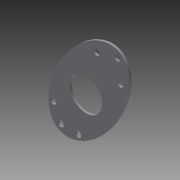
# Autodesk Inventor part: Bottom Hub Plate
Saved by Autodesk Inventor 2015 (Build 190159000, 159)
## iProperties
Created: 2015-01-24
Part Number: Bottom Hub Plate
Material: Generic
Document SubType Name: Modeling
Designer: Brian
Density: 1 g/cm^3
Appearance: Default
Author: Brian
Autodesk Inventor part; units mm, degrees
ref_plane "YZ Plane" through (0, 0, 0) normal (1, 0, 0) x (0, 1, 0)
ref_plane "XZ Plane" through (0, 0, 0) normal (0, 1, 0) x (-1, 0, 0)
ref_plane "XY Plane" through (0, 0, 0) normal (0, 0, 1) x (1, 0, 0)
sketch "Sketch1" plane through (0, 0, 0) normal (0, 0, 1) x (1, 0, 0)
  arc A0 (2.7781, 11.2277) -> (-2.7781, 11.2277) centre (0, 6.4158) ccw construction
  arc A1 (-2.7781, 11.2277) -> (-5.5562, 6.4158) centre (0, 6.4158) ccw construction
  arc A2 (-5.5562, 6.4158) -> (-2.7781, 1.604) centre (0, 6.4158) ccw construction
  arc A3 (-2.7781, 1.604) -> (2.7781, 1.604) centre (0, 6.4158) ccw construction
  arc A4 (2.7781, 1.604) -> (5.5562, 6.4158) centre (0, 6.4158) ccw construction
  arc A5 (5.5562, 6.4158) -> (2.7781, 11.2277) centre (0, 6.4158) ccw construction
  circle A6 centre (0, 6.4158) radius 3.1376 construction
  arc A7 (65.8645, 106.5408) -> (60.3083, 106.5408) centre (63.0864, 101.729) ccw construction
  arc A8 (60.3083, 106.5408) -> (57.5301, 101.729) centre (63.0864, 101.729) ccw construction
  arc A9 (57.5301, 101.729) -> (60.3083, 96.9171) centre (63.0864, 101.729) ccw construction
  arc A10 (60.3083, 96.9171) -> (65.8645, 96.9171) centre (63.0864, 101.729) ccw construction
  arc A11 (65.8645, 96.9171) -> (68.6426, 101.729) centre (63.0864, 101.729) ccw construction
  arc A12 (68.6426, 101.729) -> (65.8645, 106.5408) centre (63.0864, 101.729) ccw construction
  circle A13 centre (63.0864, 101.729) radius 3.1376 construction
  circle A14 centre (28.0384, 48.7772) radius 16.383 construction
  circle A15 centre (28.0384, 48.7772) radius 18.288
  circle A16 centre (0, 6.4158) radius 6.4158 construction
  circle A17 centre (63.0864, 101.729) radius 6.4158 construction
  circle A18 centre (63.0864, 101.729) radius 6.9238 construction
  circle A19 centre (0, 6.4158) radius 6.9238 construction
  circle A20 centre (0, 6.4158) radius 3.3916
  circle A21 centre (63.0864, 101.729) radius 3.3916
  circle A22 centre (28.0384, 48.7772) radius 38.1 construction
  line L0 (66.9079, 107.5026) -> (-3.8215, 0.6421) construction
  ellipse E0 centre (31.5432, 54.0724) end of major axis (-3.8215, 0.6421) minor radius 35.9584
  circle A23 centre (67.1501, 77.726) radius 3.302
  circle A24 centre (39.4038, 96.091) radius 3.302
  circle A25 centre (19.4364, 4.8439) radius 3.302
  circle A26 centre (-9.0413, 23.6929) radius 3.302
  line L1 (67.1501, 77.726) -> (53.277, 86.9085) construction
  line L2 (39.4038, 96.091) -> (53.277, 86.9085) construction
  line L3 (19.4364, 4.8439) -> (5.1975, 14.2684) construction
  line L4 (-9.0413, 23.6929) -> (5.1975, 14.2684) construction
  circle A27 centre (67.1501, 77.726) radius 10.5597 construction
  circle A28 centre (19.4364, 4.8439) radius 5.715 construction
  circle A29 centre (0, 6.4158) radius 13.7848 construction
  circle A30 centre (63.0864, 101.729) radius 13.7848 construction
  circle A31 centre (19.4364, 4.8439) radius 6.6675 construction
  point P0 (0, 0)
  point P1 (63.0864, 95.3131)
  point P2 (63.0864, 87.9441)
  point P3 (0, 20.2006)
  dimension "d3" = 0.508
  dimension "d4" = 0.508
  dimension "d0" = 1.905
  dimension "d1" = 0.254
  dimension "d2" = 0.254
  dimension "d6" = 6.604
  dimension "d7" = 6.604
  dimension "d8" = 6.604
  dimension "d9" = 6.604
  dimension "d12" = 11.43
  dimension "d13" = 13.335
  constraints: 12 coincident, 10 centre point, 10 end point, 5 point on line, 4 collinear, 4 vertical alignment, 2 tangent, 1 midpoint, 1 parallel, 1 perpendicular, 26 other
  measures "d0" radial gap between concentric circles of A15 A14
  measures "d1" radial gap between concentric circles of A13 A21
  measures "d2" radial gap between concentric circles of A6 A20
  measures "d6" diameter of A23
  measures "d7" diameter of A24
  measures "d8" diameter of A25
  measures "d9" diameter of A26
  measures "d12" diameter of A28
  measures "d13" diameter of A31
extrude "Extrusion1" add sketch "Sketch1" along normal blind 2.2733
equation "\"d2\" = d1"
equation "\"d7\" = d6"
equation "\"d8\" = d6"
equation "\"d9\" = d6"
body "Solid1"
